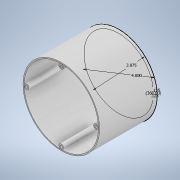
# Autodesk Inventor part: Main Iris box
Saved by Autodesk Inventor 2021 (Build 250183000, 183)
## iProperties
Created: 2020-07-09
Part Number: Main Iris box
Material: Generic
Document SubType Name: Modeling
Designer: saipr
Density: 1 g/cm^3
Appearance: Default
Author: saipr
Autodesk Inventor part; units mm, degrees
ref_plane "YZ Plane" through (0, 0, 0) normal (1, 0, 0) x (0, 1, 0)
ref_plane "XZ Plane" through (0, 0, 0) normal (0, 1, 0) x (-1, 0, 0)
ref_plane "XY Plane" through (0, 0, 0) normal (0, 0, 1) x (1, 0, 0)
sketch "Sketch1" plane through (0, 0, 0) normal (0, 0, 1) x (1, 0, 0)
  circle A0 centre (0, 0) radius 50.8
  circle A1 centre (0, 0) radius 49.2125
  line L0 (49.2125, 0) -> (46.0375, 0)
  circle A2 centre (46.0375, 0) radius 3.175
  circle A3 centre (46.0375, 0) radius 1.5875
  circle A4 centre (0, 46.0375) radius 1.5875
  circle A5 centre (0, 46.0375) radius 3.175
  circle A6 centre (-46.0375, 0) radius 1.5875
  circle A7 centre (-46.0375, 0) radius 3.175
  circle A8 centre (0, -46.0375) radius 1.5875
  circle A9 centre (0, -46.0375) radius 3.175
  point P0 (0, 49.2125)
  point P1 (-49.2125, 0)
  point P2 (0, -49.2125)
  point P3 (0, 49.2125)
  point P4 (0, -49.2125)
  point P5 (-49.2125, 0)
  dimension "d1" = 98.425
  dimension "d0" = 101.6
  dimension "d6" = 3.175
  dimension "d7" = 3.175
  dimension "d10" = 360
  constraints: 7 coincident, 5 centre point, 2 end point, 1 horizontal, 1 horizontal alignment, 35 other
  measures "d0" diameter of A0
  measures "d6" distance of L0.start L0.end
  measures "d7" diameter of A3
extrude "Extrusion1" add sketch "Sketch1" along normal blind 6.35 contours A5 | A7 | A9 | A1 | A2 | A3 | A4 | A6 | A8
extrude "Extrusion3" add sketch "Sketch1" along normal blind 76.2
body "Solid1"
